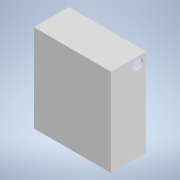
# Autodesk Inventor part: corpo
Saved by Autodesk Inventor 2020 (Build 240168000, 168)
## iProperties
Created: 2021-03-19
Part Number: corpo
Material: Generic
Document SubType Name: Modeling
Designer: super
Density: 1 g/cm^3
Appearance: Default
Author: super
Autodesk Inventor part; units mm, degrees
ref_plane "YZ Plane" through (0, 0, 0) normal (1, 0, 0) x (0, 1, 0)
ref_plane "XZ Plane" through (0, 0, 0) normal (0, 1, 0) x (-1, 0, 0)
ref_plane "XY Plane" through (0, 0, 0) normal (0, 0, 1) x (1, 0, 0)
sketch "Sketch1" plane through (0, 0, 0) normal (0, 0, 1) x (1, 0, 0)
  line L0 (0, 0) -> (220, 0)
  line L1 (220, 0) -> (220, 250)
  line L2 (220, 250) -> (0, 250)
  line L3 (0, 250) -> (0, 0)
  dimension "d0" = 220
  dimension "d1" = 250
  constraints: 8 end point, 2 parallel, 1 horizontal, 1 perpendicular
  measures "d0" distance of L2.end L1.end
  measures "d1" distance of L1.end L0.end
extrude "Extrusion1" add sketch "Sketch1" along normal blind 100
sketch "Sketch2" plane through (0, 0, 0) normal (0, 0, 1) x (1, 0, 0)
  line L0 (5, 5) -> (215, 5)
  line L1 (215, 5) -> (215, 245)
  line L2 (215, 245) -> (5, 245)
  line L3 (5, 245) -> (5, 5)
  point P0 (0, 0)
  dimension "d4" = 210
  dimension "d5" = 240
  dimension "d8" = 5
  dimension "d13" = 5
  constraints: 8 end point, 2 parallel, 1 horizontal, 1 perpendicular
  measures "d4" distance of L2.end L1.end
  measures "d5" distance of L1.end L0.end
  measures "d8" horizontal distance of point (0, 0) L0.start
  measures "d13" horizontal distance of point (0, 0) L0.start
extrude "Extrusion2" cut sketch "Sketch2" along normal blind 95
sketch "Sketch3" plane through (220, 0, 0) normal (1, 0, 0) x (0, 0, -1)
  circle A0 centre (-23.8569, 230) radius 15
  line L0 (0, 250) -> (-100, 250) projected
  point P0 (0, 0)
  dimension "d9" = 30
  dimension "d10" = 20
  constraints: 1 centre point
  measures "d9" diameter of A0
  measures "d10" distance from line of L0 A0.centre
extrude "Extrusion3" cut sketch "Sketch3" against normal blind 45
sketch "Sketch4" plane through (0, 0, 0) normal (-1, 0, 0) x (0, 0, 1)
  circle A0 centre (73.7116, 232.2043) radius 14.7089
  point P0 (0, 0)
  constraints: 1 centre point
extrude "Extrusion4" cut sketch "Sketch4" against normal blind 10
body "Solid1"
